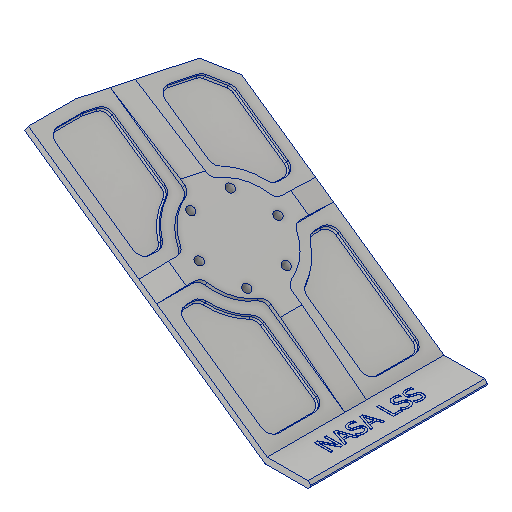
# Autodesk Inventor part: CNCM_ALU_Sorting_shovel_top_plate
Saved by Autodesk Inventor 2025 (Build 290162010, 162A)
## iProperties
Created: 2018-09-12
Part Number: CNCM_ALU_Sorting_shovel_top_plate
Material: Aluminum 6061
Document SubType Name: Modeling
Designer: Andrzej
Density: 2.7 g/cm^3
Appearance: Aluminum - Flat
Mass: 46.5168 g
Surface Area: 175.12 cm^2
Volume: 17.2284 cm^3
Author: Andrzej
Autodesk Inventor part; units mm, degrees
ref_plane "YZ Plane" through (0, 0, 0) normal (1, 0, 0) x (0, 1, 0)
ref_plane "XZ Plane" through (0, 0, 0) normal (0, 1, 0) x (-1, 0, 0)
ref_plane "XY Plane" through (0, 0, 0) normal (0, 0, 1) x (1, 0, 0)
sketch "Sketch3" plane through (0, 0, 0) normal (0, 0, 1) x (1, 0, 0)
  line L0 (-22.236, -1.7566) -> (-6.236, -1.7566)
  line L1 (-22.236, -1.7566) -> (-111.7161, 60.898)
  line L2 (-6.236, -4.2566) -> (-6.236, -1.7566)
  line L3 (-6.236, -4.2566) -> (-23.0242, -4.2566)
  line L4 (-23.0242, -4.2566) -> (-113.15, 58.8501)
  line L5 (-111.7161, 60.898) -> (-113.15, 58.8501)
  point P0 (0, 0)
  dimension "d20" = 2.5
  dimension "d21" = 16
  dimension "d22" = 145
  dimension "d23" = 109.2351
  dimension "d24" = 2.5
  constraints: 12 end point, 2 horizontal
  measures "d20" distance between parallel lines of L1 L4
  measures "d21" distance of L0.start L0.end
  measures "d22" angle of L1 L0
  measures "d23" distance of L0.start L1.end
  measures "d24" distance between parallel lines of L3 L0
extrude "Extrusion4" add sketch "Sketch3" along normal blind 65
sketch "Sketch4" plane through (-111.7161, 60.898, 65) normal (0.5735764, 0.819152, 0) x (0.819152, -0.5735764, 0)
  line L0 (109.2351, 65) -> (0, 65) projected
  line L1 (0, 65) -> (0, 0) projected
  line L2 (109.2351, 0) -> (0, 0) projected
  line L3 (109.2351, 65) -> (109.2351, 0) projected
  line L4 (0, 65) -> (0, 0) projected
  line L5 (0, 17.5) -> (8.3755, 65)
  line L6 (2, 0) -> (2, 17.325)
  line L7 (2, 17.325) -> (10.4064, 65)
  point P0 (126.4421, 65)
  dimension "d27" = 17.5
  dimension "d28" = 170
  dimension "d31" = 2
  dimension "d32" = 2
  constraints: 6 end point, 4 point on line, 1 parallel, 1 vertical
  measures "d27" distance from line of L5.start L2
  measures "d28" angle of L1 L5
  measures "d31" distance between parallel lines of L1 L6
  measures "d32" distance between parallel lines of L5 L7
extrude "Extrusion5" cut sketch "Sketch4" against normal blind 65 contours L7 L6 L2 L1 L5 L0 | L5 L1 L0
chamfer "Chamfer1" distance 8 angle 45 1 edges at (-103.9086, 53.9052, 0)
sketch "Sketch6" plane through (-22.236, -1.7566, 65) normal (0.5735764, 0.819152, 0) x (0.819152, -0.5735764, 0)
  line L0 (0, 65) -> (0, 0) projected
  line L1 (-107.2351, 17.325) -> (-107.2351, 0) projected
  line L2 (-100.2179, 57.1215) -> (-90.8287, 65) projected
  line L3 (-100.2179, 57.1215) -> (-107.2351, 17.325) projected
  line L4 (-107.2351, 17.325) -> (-107.2351, 0) projected
  line L5 (0, 0) -> (-107.2351, 0) projected
  line L6 (0, 65) -> (0, 0) projected
  line L7 (0, 65) -> (-90.8287, 65) projected
  circle A0 centre (-53.6175, 32.5) radius 17.5
  line L8 (-57.6175, 0) -> (-57.6175, 15.4633)
  line L9 (-49.6175, 0) -> (-49.6175, 15.4633)
  line L10 (-36.5808, 28.5) -> (0, 28.5)
  line L11 (-36.5808, 36.5) -> (0, 36.5)
  line L12 (-49.6175, 49.5367) -> (-49.6175, 65)
  line L13 (-57.6175, 49.5367) -> (-57.6175, 65)
  line L14 (-103.854, 36.5) -> (-70.6543, 36.5)
  line L15 (-105.2646, 28.5) -> (-70.6543, 28.5)
  point P0 (17.2071, 65)
  dimension "d41" = 35
  dimension "d39" = 107.2351
  dimension "d40" = 65
  dimension "d42" = 32.5
  dimension "d43" = 53.6175
  dimension "d45" = 4
  dimension "d46" = 4
  dimension "d47" = 4
  dimension "d48" = 4
  constraints: 16 end point, 8 point on line, 4 collinear, 4 perpendicular, 4 vertical, 10 other
  measures "d39" distance between parallel lines of L0 L1
  measures "d40" distance between parallel lines of L7 L5
  measures "d42" distance from line of L5 point (-53.618, 32.5)
  measures "d43" distance from line of L1 point (-53.618, 32.5)
  measures "d45" distance from line of point (-53.618, 32.5) L8
  measures "d46" distance from line of point (-53.618, 32.5) L9
  measures "d47" distance from line of point (-53.618, 32.5) L15
  measures "d48" distance from line of point (-53.618, 32.5) L14
extrude "Extrusion7" add sketch "Sketch6" along normal blind 1.5 contours L0 L10 A0 L11 | L12 A0 L13 L7 | A0 | L5 L8 A0 L9 | A0 L15 L3 L14
sketch "Sketch7" plane through (-110.0778, 59.7509, 65) normal (0.5735764, 0.819152, 0) x (0.819152, -0.5735764, 0)
  line L0 (70.6543, 36.5) -> (107.2351, 36.5) projected
  line L1 (107.2351, 65) -> (107.2351, 36.5) projected
  line L2 (107.2351, 65) -> (57.6175, 65) projected
  line L3 (57.6175, 65) -> (57.6175, 49.5367) projected
  arc A0 (70.6543, 36.5) -> (57.6175, 49.5367) centre (53.6175, 32.5) ccw projected
  line L4 (49.6175, 49.5367) -> (49.6175, 65) projected
  line L5 (49.6175, 65) -> (16.4064, 65) projected
  line L6 (7.0172, 57.1215) -> (16.4064, 65) projected
  line L7 (7.0172, 57.1215) -> (3.3811, 36.5) projected
  line L8 (3.3811, 36.5) -> (36.5808, 36.5) projected
  arc A1 (49.6175, 49.5367) -> (36.5808, 36.5) centre (53.6175, 32.5) ccw projected
  line L9 (107.2351, 28.5) -> (70.6543, 28.5) projected
  arc A2 (57.6175, 15.4633) -> (70.6543, 28.5) centre (53.6175, 32.5) ccw projected
  line L10 (57.6175, 15.4633) -> (57.6175, 0) projected
  line L11 (107.2351, 0) -> (57.6175, 0) projected
  line L12 (107.2351, 28.5) -> (107.2351, 0) projected
  line L13 (49.6175, 0) -> (49.6175, 15.4633) projected
  arc A3 (36.5808, 28.5) -> (49.6175, 15.4633) centre (53.6175, 32.5) ccw projected
  line L14 (36.5808, 28.5) -> (1.9705, 28.5) projected
  line L15 (1.9705, 28.5) -> (0, 17.325) projected
  line L16 (0, 17.325) -> (0, 0) projected
  line L17 (49.6175, 0) -> (0, 0) projected
  line L18 (17.8623, 61) -> (45.6175, 61)
  line L19 (45.6175, 61) -> (45.6175, 52.4562)
  arc A4 (45.6175, 52.4562) -> (33.6613, 40.5) centre (53.6175, 32.5) ccw
  line L20 (33.6613, 40.5) -> (8.1481, 40.5)
  line L21 (8.1481, 40.5) -> (10.7036, 54.9932)
  line L22 (10.7036, 54.9932) -> (17.8623, 61)
  line L23 (5.3268, 24.5) -> (33.6613, 24.5)
  arc A5 (33.6613, 24.5) -> (45.6175, 12.5438) centre (53.6175, 32.5) ccw
  line L24 (45.6175, 12.5438) -> (45.6175, 4)
  line L25 (45.6175, 4) -> (4, 4)
  line L26 (4, 4) -> (4, 16.9751)
  line L27 (4, 16.9751) -> (5.3268, 24.5)
  line L28 (73.5737, 24.5) -> (103.2351, 24.5)
  line L29 (103.2351, 24.5) -> (103.2351, 4)
  line L30 (103.2351, 4) -> (61.6175, 4)
  line L31 (61.6175, 4) -> (61.6175, 12.5438)
  arc A6 (61.6175, 12.5438) -> (73.5737, 24.5) centre (53.6175, 32.5) ccw
  line L32 (103.2351, 40.5) -> (73.5737, 40.5)
  arc A7 (73.5737, 40.5) -> (61.6175, 52.4562) centre (53.6175, 32.5) ccw
  line L33 (61.6175, 52.4562) -> (61.6175, 61)
  line L34 (61.6175, 61) -> (103.2351, 61)
  line L35 (103.2351, 61) -> (103.2351, 40.5)
  point P0 (124.4421, 65)
  dimension "d51" = 4
  dimension "d52" = 4
  dimension "d53" = 4
  dimension "d54" = 4
  constraints: 36 end point, 8 point on circle, 4 centre point, 18 other
  measures "d51" distance between parallel lines of L5 L18
  measures "d52" distance between parallel lines of L14 L23
  measures "d53" radial gap between concentric circles of A2 A6
  measures "d54" distance between parallel lines of L0 L32
extrude "Extrusion8" cut sketch "Sketch7" against normal blind 1.5 contours L18 L19 A4 L20 L21 L22 | L23 A5 L24 L25 L26 L27 | L28 L29 L30 L31 A6 | L32 A7 L33 L34 L35
chamfer "Chamfer2" distance 30 distance2 1.5 1 edges at (-107.0256, 59.4448, 32.5) measured on face at (-68.6742, 32.591, 30.0745)
chamfer "Chamfer3" distance 30 distance2 1.5 1 edges at (-21.3756, -0.5279, 32.5) measured on face at (-67.3858, 31.6888, 27.2538)
chamfer "Chamfer4" distance 10 distance2 1.5 1 edges at (-65.2965, 30.2258, 65) measured on face at (-63.2072, 28.7629, 37.7462)
chamfer "Chamfer5" distance 10 distance2 1.5 1 edges at (-65.2965, 30.2258, 0) measured on face at (-69.0287, 32.8392, 28.8573)
sketch "Sketch8" plane through (-21.3756, -0.5279, 65) normal (0.5735764, 0.819152, 0) x (0.819152, -0.5735764, 0)
  line L0 (-57.6175, 55) -> (-49.6175, 55) projected
  line L1 (-57.6175, 55) -> (-57.6175, 49.5367) projected
  arc A0 (-57.6175, 49.5367) -> (-70.6543, 36.5) centre (-53.6175, 32.5) ccw projected
  line L2 (-70.6543, 36.5) -> (-73.3912, 36.5) projected
  line L3 (-74.8018, 28.5) -> (-73.3912, 36.5) projected
  line L4 (-74.8018, 28.5) -> (-70.6543, 28.5) projected
  arc A1 (-70.6543, 28.5) -> (-57.6175, 15.4633) centre (-53.6175, 32.5) ccw projected
  line L5 (-57.6175, 15.4633) -> (-57.6175, 10) projected
  line L6 (-49.6175, 10) -> (-57.6175, 10) projected
  line L7 (-49.6175, 10) -> (-49.6175, 15.4633) projected
  arc A2 (-49.6175, 15.4633) -> (-36.5808, 28.5) centre (-53.6175, 32.5) ccw projected
  line L8 (-36.5808, 28.5) -> (-30, 28.5) projected
  line L9 (-30, 36.5) -> (-30, 28.5) projected
  line L10 (-30, 36.5) -> (-36.5808, 36.5) projected
  arc A3 (-36.5808, 36.5) -> (-49.6175, 49.5367) centre (-53.6175, 32.5) ccw projected
  line L11 (-49.6175, 49.5367) -> (-49.6175, 55) projected
  circle A4 centre (-53.6175, 47) radius 1.5
  circle A5 centre (-53.6175, 32.5) radius 17.5
  circle A6 centre (-66.1749, 39.75) radius 1.5
  circle A7 centre (-66.1749, 25.25) radius 1.5
  circle A8 centre (-53.6175, 18) radius 1.5
  circle A9 centre (-41.0602, 25.25) radius 1.5
  circle A10 centre (-41.0602, 39.75) radius 1.5
  point P0 (17.2071, 65)
  dimension "d69" = 3
  dimension "d70" = 14.5
  dimension "d73" = 360
  constraints: 7 centre point, 1 coincident, 1 concentric, 13 other
  measures "d69" diameter of A4
  measures "d70" distance of A4.centre A0.centre
extrude "Extrusion9" cut sketch "Sketch8" against normal through all contours A4 | A6 | A7 | A8 | A9 | A10
fillet "Fillet2" radius 3.5 22 edges at (-106.145, 56.0803, 40.5) (-82.9348, 39.8283, 40.5) (-73.1408, 32.9705, 52.4562) (-107.2319, 56.8414, 61) (-73.1408, 32.9705, 61) (-103.834, 54.4621, 24.5) (-101.7406, 52.9963, 10.0068) (-95.8766, 48.8903, 4) (-73.1408, 32.9705, 4) (-73.1408, 32.9705, 12.5438) (-82.9348, 39.8283, 24.5) (-60.0344, 23.7933, 12.5438) (-60.0344, 23.7933, 4) (-50.2405, 16.9355, 24.5) (-25.9433, -0.0775, 24.5) (-25.9433, -0.0775, 4) (-25.9433, -0.0775, 40.5) (-25.9433, -0.0775, 61) (-50.2405, 16.9355, 40.5) (-60.0344, 23.7933, 52.4562) (-60.0344, 23.7933, 61) (-107.2319, 56.8414, 48.0249)
fillet "Fillet3" radius 0.5 44 edges at (-83.7121, 39.4558, 41.0096) (-79.4718, 36.4867, 47.7028) (-73.989, 32.6477, 52.8793) (-73.5716, 32.3554, 56.099) (-74.4113, 32.9434, 59.9749) (-90.6171, 44.2908, 61) (-106.8229, 55.6382, 59.9749) (-107.6627, 56.2262, 52.9156) (-107.6518, 56.2186, 48.0261) (-107.3063, 55.9767, 45.5578) (-106.0129, 55.071, 41.3188) (-94.686, 47.1398, 40.5) (-96.2444, 48.2311, 4.2111) (-85.8512, 40.9537, 4) (-74.4113, 32.9434, 5.0251) (-73.5716, 32.3554, 8.901) (-73.989, 32.6477, 12.1207) (-79.4718, 36.4867, 17.2972) (-83.7121, 39.4558, 23.9904) (-93.0249, 45.9767, 24.5) (-103.0442, 52.9923, 23.2498) (-103.012, 52.9698, 15.8268) (-102.012, 52.2696, 10.1191) (-99.2394, 50.3281, 7.0034) (-27.2138, -0.1047, 5.0251) (-26.3741, -0.6927, 14.25) (-27.2138, -0.1047, 23.4749) (-39.038, 8.1747, 24.5) (-50.3246, 16.0777, 23.9904) (-54.565, 19.0468, 17.2972) (-60.0477, 22.8858, 12.1207) (-60.4652, 23.1781, 8.901) (-59.6254, 22.5902, 5.0251) (-43.4196, 11.2427, 4) (-27.2138, -0.1047, 41.5251) (-26.3741, -0.6927, 50.75) (-27.2138, -0.1047, 59.9749) (-43.4196, 11.2427, 61) (-59.6254, 22.5902, 59.9749) (-60.4652, 23.1781, 56.099) (-60.0477, 22.8858, 52.8793) (-54.565, 19.0468, 47.7028) (-50.3246, 16.0777, 41.0096) (-39.038, 8.1747, 40.5)
fillet "Fillet4" radius 3 8 edges at (-79.6823, 39.3833, 36.5) (-69.0033, 31.9058, 49.5367) (-62.4501, 27.3172, 49.5367) (-51.771, 19.8396, 36.5) (-51.771, 19.8396, 28.5) (-62.4501, 27.3172, 15.4633) (-69.0033, 31.9058, 15.4633) (-79.6823, 39.3833, 28.5)
chamfer "Chamfer6" distance 1 angle 45 2 edges at (-6.236, -1.7566, 32.5) (-6.236, -4.2566, 32.5)
sketch "Sketch9" plane through (-22.236, -1.7566, 28.5) normal (0, 1, 0) x (1, 0, 0)
  line L0 (15, 28.5) -> (15, -36.5) projected
  line L1 (15, 28.5) -> (0, 28.5) projected
  line L2 (0, 28.5) -> (0, 0) projected
  line L3 (0, 0) -> (0, -8) projected
  line L4 (0, -8) -> (0, -36.5) projected
  line L5 (15, -36.5) -> (0, -36.5) projected
  line L6 (3.9426, -23.8151) -> (3.9426, 23.433) construction
  line L7 (3.9426, 23.433) -> (13.0769, 23.433) construction
  line L8 (13.0769, 23.433) -> (13.0769, -23.8151) construction
  line L9 (13.0769, -23.8151) -> (3.9426, -23.8151) construction
  line L10 (10.1514, -18.8323) -> (10.1514, -19.7419)
  line L11 (10.1514, -19.7419) -> (4.8917, -22.4409)
  line L12 (4.8917, -22.4409) -> (10.1514, -22.4409)
  line L13 (10.1514, -22.4409) -> (10.1514, -23.1972)
  line L14 (10.1514, -23.1972) -> (4.0514, -23.1972)
  line L15 (4.0514, -23.1972) -> (4.0514, -22.0455)
  line L16 (4.0514, -22.0455) -> (8.881, -19.5886)
  line L17 (8.881, -19.5886) -> (4.0514, -19.5886)
  line L18 (4.0514, -19.5886) -> (4.0514, -18.8323)
  line L19 (4.0514, -18.8323) -> (10.1514, -18.8323)
  line L20 (10.1514, -18.254) -> (4.0514, -16.1976)
  line L21 (4.0514, -16.1976) -> (4.0514, -15.199)
  line L22 (4.0514, -15.199) -> (10.1514, -13.1426)
  line L23 (10.1514, -13.1426) -> (10.1514, -13.9978)
  line L24 (10.1514, -13.9978) -> (8.446, -14.5514)
  line L25 (8.446, -14.5514) -> (8.446, -16.8797)
  line L26 (8.446, -16.8797) -> (10.1514, -17.4334)
  line L27 (10.1514, -17.4334) -> (10.1514, -18.254)
  line L28 (7.7539, -14.7739) -> (4.8819, -15.7181)
  line L29 (4.8819, -15.7181) -> (7.7539, -16.6573)
  line L30 (7.7539, -16.6573) -> (7.7539, -14.7739)
  spline S0 degree 2 poles (10.2601, -10.8638) (10.2601, -11.5262) (9.9833, -12.4555) (9.7856, -12.8658) knots 0 0 0 1 2 2 2
  line L31 (9.7856, -12.8658) -> (8.7673, -12.8658)
  line L32 (8.7673, -12.8658) -> (8.7673, -12.8065)
  spline S1 degree 2 poles (8.7673, -12.8065) (9.143, -12.4061) (9.5582, -11.3927) (9.5582, -10.9231) knots 0 0 0 1 2 2 2
  spline S2 degree 2 poles (9.5582, -10.9231) (9.5582, -10.2508) (8.9996, -9.5637) (8.5399, -9.5637) knots 0 0 0 1 2 2 2
  spline S3 degree 2 poles (8.5399, -9.5637) (8.1741, -9.5637) (7.7193, -9.9245) (7.6056, -10.3151) knots 0 0 0 1 2 2 2
  spline S4 degree 2 poles (7.6056, -10.3151) (7.5265, -10.5968) (7.4178, -11.0664) (7.3288, -11.4174) knots 0 0 0 1 2 2 2
  spline S5 degree 2 poles (7.3288, -11.4174) (7.2447, -11.7338) (6.9926, -12.2331) (6.79, -12.4258) knots 0 0 0 1 2 2 2
  spline S6 degree 2 poles (6.79, -12.4258) (6.5873, -12.6137) (6.0435, -12.8213) (5.6876, -12.8213) knots 0 0 0 1 2 2 2
  spline S7 degree 2 poles (5.6876, -12.8213) (4.9461, -12.8213) (3.9426, -11.6646) (3.9426, -10.7698) knots 0 0 0 1 2 2 2
  spline S8 degree 2 poles (3.9426, -10.7698) (3.9426, -10.2557) (4.1453, -9.3462) (4.3381, -8.9557) knots 0 0 0 1 2 2 2
  line L33 (4.3381, -8.9557) -> (5.307, -8.9557)
  line L34 (5.307, -8.9557) -> (5.307, -9.015)
  spline S9 degree 2 poles (5.307, -9.015) (5.04, -9.3066) (4.6446, -10.2162) (4.6446, -10.7155) knots 0 0 0 1 2 2 2
  spline S10 degree 2 poles (4.6446, -10.7155) (4.6446, -11.279) (5.1735, -11.976) (5.6036, -11.976) knots 0 0 0 1 2 2 2
  spline S11 degree 2 poles (5.6036, -11.976) (5.9892, -11.976) (6.4489, -11.5657) (6.5527, -11.1801) knots 0 0 0 1 2 2 2
  spline S12 degree 2 poles (6.5527, -11.1801) (6.6219, -10.9231) (6.7999, -10.1767) (6.874, -9.9295) knots 0 0 0 1 2 2 2
  spline S13 degree 2 poles (6.874, -9.9295) (7.0668, -9.3017) (7.8429, -8.7184) (8.4114, -8.7184) knots 0 0 0 1 2 2 2
  spline S14 degree 2 poles (8.4114, -8.7184) (8.7722, -8.7184) (9.4643, -9.01) (9.7065, -9.272) knots 0 0 0 1 2 2 2
  spline S15 degree 2 poles (9.7065, -9.272) (9.9734, -9.5637) (10.2601, -10.3052) (10.2601, -10.8638) knots 0 0 0 1 2 2 2
  line L35 (10.1514, -8.5503) -> (4.0514, -6.4939)
  line L36 (4.0514, -6.4939) -> (4.0514, -5.4954)
  line L37 (4.0514, -5.4954) -> (10.1514, -3.439)
  line L38 (10.1514, -3.439) -> (10.1514, -4.2942)
  line L39 (10.1514, -4.2942) -> (8.446, -4.8478)
  line L40 (8.446, -4.8478) -> (8.446, -7.1761)
  line L41 (8.446, -7.1761) -> (10.1514, -7.7297)
  line L42 (10.1514, -7.7297) -> (10.1514, -8.5503)
  line L43 (7.7539, -5.0703) -> (4.8819, -6.0144)
  line L44 (4.8819, -6.0144) -> (7.7539, -6.9536)
  line L45 (7.7539, -6.9536) -> (7.7539, -5.0703)
  line L46 (10.1514, 3.2938) -> (10.1514, -0.2407)
  line L47 (10.1514, -0.2407) -> (4.0514, -0.2407)
  line L48 (4.0514, -0.2407) -> (4.0514, 0.57)
  line L49 (4.0514, 0.57) -> (9.4297, 0.57)
  line L50 (9.4297, 0.57) -> (9.4297, 3.2938)
  line L51 (9.4297, 3.2938) -> (10.1514, 3.2938)
  spline S16 degree 2 poles (10.2601, 5.6319) (10.2601, 4.9695) (9.9833, 4.0402) (9.7856, 3.6299) knots 0 0 0 1 2 2 2
  line L52 (9.7856, 3.6299) -> (8.7673, 3.6299)
  line L53 (8.7673, 3.6299) -> (8.7673, 3.6892)
  spline S17 degree 2 poles (8.7673, 3.6892) (9.143, 4.0896) (9.5582, 5.103) (9.5582, 5.5726) knots 0 0 0 1 2 2 2
  spline S18 degree 2 poles (9.5582, 5.5726) (9.5582, 6.2449) (8.9996, 6.932) (8.5399, 6.932) knots 0 0 0 1 2 2 2
  spline S19 degree 2 poles (8.5399, 6.932) (8.1741, 6.932) (7.7193, 6.5712) (7.6056, 6.1806) knots 0 0 0 1 2 2 2
  spline S20 degree 2 poles (7.6056, 6.1806) (7.5265, 5.8989) (7.4178, 5.4293) (7.3288, 5.0783) knots 0 0 0 1 2 2 2
  spline S21 degree 2 poles (7.3288, 5.0783) (7.2447, 4.7619) (6.9926, 4.2627) (6.79, 4.0699) knots 0 0 0 1 2 2 2
  spline S22 degree 2 poles (6.79, 4.0699) (6.5873, 3.882) (6.0435, 3.6744) (5.6876, 3.6744) knots 0 0 0 1 2 2 2
  spline S23 degree 2 poles (5.6876, 3.6744) (4.9461, 3.6744) (3.9426, 4.8311) (3.9426, 5.7259) knots 0 0 0 1 2 2 2
  spline S24 degree 2 poles (3.9426, 5.7259) (3.9426, 6.24) (4.1453, 7.1495) (4.3381, 7.54) knots 0 0 0 1 2 2 2
  line L54 (4.3381, 7.54) -> (5.307, 7.54)
  line L55 (5.307, 7.54) -> (5.307, 7.4807)
  spline S25 degree 2 poles (5.307, 7.4807) (5.04, 7.1891) (4.6446, 6.2795) (4.6446, 5.7802) knots 0 0 0 1 2 2 2
  spline S26 degree 2 poles (4.6446, 5.7802) (4.6446, 5.2167) (5.1735, 4.5197) (5.6036, 4.5197) knots 0 0 0 1 2 2 2
  spline S27 degree 2 poles (5.6036, 4.5197) (5.9892, 4.5197) (6.4489, 4.93) (6.5527, 5.3156) knots 0 0 0 1 2 2 2
  spline S28 degree 2 poles (6.5527, 5.3156) (6.6219, 5.5726) (6.7999, 6.3191) (6.874, 6.5662) knots 0 0 0 1 2 2 2
  spline S29 degree 2 poles (6.874, 6.5662) (7.0668, 7.194) (7.8429, 7.7773) (8.4114, 7.7773) knots 0 0 0 1 2 2 2
  spline S30 degree 2 poles (8.4114, 7.7773) (8.7722, 7.7773) (9.4643, 7.4857) (9.7065, 7.2237) knots 0 0 0 1 2 2 2
  spline S31 degree 2 poles (9.7065, 7.2237) (9.9734, 6.932) (10.2601, 6.1905) (10.2601, 5.6319) knots 0 0 0 1 2 2 2
  spline S32 degree 2 poles (10.2601, 10.3033) (10.2601, 9.6409) (9.9833, 8.7116) (9.7856, 8.3013) knots 0 0 0 1 2 2 2
  line L56 (9.7856, 8.3013) -> (8.7673, 8.3013)
  line L57 (8.7673, 8.3013) -> (8.7673, 8.3606)
  spline S33 degree 2 poles (8.7673, 8.3606) (9.143, 8.761) (9.5582, 9.7744) (9.5582, 10.244) knots 0 0 0 1 2 2 2
  spline S34 degree 2 poles (9.5582, 10.244) (9.5582, 10.9163) (8.9996, 11.6034) (8.5399, 11.6034) knots 0 0 0 1 2 2 2
  spline S35 degree 2 poles (8.5399, 11.6034) (8.1741, 11.6034) (7.7193, 11.2426) (7.6056, 10.852) knots 0 0 0 1 2 2 2
  spline S36 degree 2 poles (7.6056, 10.852) (7.5265, 10.5703) (7.4178, 10.1007) (7.3288, 9.7497) knots 0 0 0 1 2 2 2
  spline S37 degree 2 poles (7.3288, 9.7497) (7.2447, 9.4333) (6.9926, 8.934) (6.79, 8.7413) knots 0 0 0 1 2 2 2
  spline S38 degree 2 poles (6.79, 8.7413) (6.5873, 8.5534) (6.0435, 8.3458) (5.6876, 8.3458) knots 0 0 0 1 2 2 2
  spline S39 degree 2 poles (5.6876, 8.3458) (4.9461, 8.3458) (3.9426, 9.5025) (3.9426, 10.3973) knots 0 0 0 1 2 2 2
  spline S40 degree 2 poles (3.9426, 10.3973) (3.9426, 10.9114) (4.1453, 11.8209) (4.3381, 12.2114) knots 0 0 0 1 2 2 2
  line L58 (4.3381, 12.2114) -> (5.307, 12.2114)
  line L59 (5.307, 12.2114) -> (5.307, 12.1521)
  spline S41 degree 2 poles (5.307, 12.1521) (5.04, 11.8605) (4.6446, 10.9509) (4.6446, 10.4516) knots 0 0 0 1 2 2 2
  spline S42 degree 2 poles (4.6446, 10.4516) (4.6446, 9.8881) (5.1735, 9.1911) (5.6036, 9.1911) knots 0 0 0 1 2 2 2
  spline S43 degree 2 poles (5.6036, 9.1911) (5.9892, 9.1911) (6.4489, 9.6014) (6.5527, 9.987) knots 0 0 0 1 2 2 2
  spline S44 degree 2 poles (6.5527, 9.987) (6.6219, 10.244) (6.7999, 10.9904) (6.874, 11.2376) knots 0 0 0 1 2 2 2
  spline S45 degree 2 poles (6.874, 11.2376) (7.0668, 11.8654) (7.8429, 12.4487) (8.4114, 12.4487) knots 0 0 0 1 2 2 2
  spline S46 degree 2 poles (8.4114, 12.4487) (8.7722, 12.4487) (9.4643, 12.1571) (9.7065, 11.8951) knots 0 0 0 1 2 2 2
  spline S47 degree 2 poles (9.7065, 11.8951) (9.9734, 11.6034) (10.2601, 10.8619) (10.2601, 10.3033) knots 0 0 0 1 2 2 2
  point P0 (22.236, 28.5)
  constraints: 2 other
extrude "Extrusion10" cut sketch "Sketch9" against normal blind 0.1 contours L10 L11 L12 L13 L14 L15 L16 L17 L18 L19 | L20 L21 L22 L23 L24 L25 L26 L27 | S0 L31 L32 S1 S2 S3 S4 S5 S6 S7 S8 L33 L34 S9 S10 S11 S12 S13 S14 S15 | L35 L36 L37 L38 L39 L40 L41 L42 | L46 L47 L48 L49 L50 L51 | S16 L52 L53 S17 S18 S19 S20 S21 S22 S23 S24 L54 L55 S25 S26 S27 S28 S29 S30 S31 | S32 L56 L57 S33 S34 S35 S36 S37 S38 S39 S40 L58 L59 S41 S42 S43 S44 S45 S46 S47
equation "\"d20\" = d19"
equation "\"d32\" = d31"
equation "\"d42\" = 0.5 * d40"
equation "\"d43\" = 0.5 * d39"
equation "\"d46\" = d45"
equation "\"d48\" = d47"
equation "\"d19\" = 2.5"
body "Solid2"
